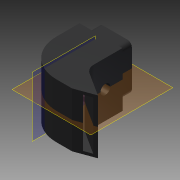
# Autodesk Inventor part: Tobera_05
Saved by Autodesk Inventor 2015 (Build 190159000, 159)
## iProperties
Created: 2013-03-26
Part Number: Tobera_05
Document SubType Name: Modeling
Designer: Lukas
Density: 1 g/cm^3
Mass: 3.92133 g
Surface Area: 46.33 cm^2
Volume: 3.92133 cm^3
Material: Generic
Appearance: Rubber - Black - Version 1.1
Author: Lukas
Autodesk Inventor part; units mm, degrees
ref_plane "YZ Plane" through (0, 0, 0) normal (1, 0, 0) x (0, 1, 0)
ref_plane "XZ Plane" through (0, 0, 0) normal (0, 1, 0) x (-1, 0, 0)
sketch "Boceto1" plane through (0, 0, 0) normal (0, 0, 1) x (1, 0, 0)
  line L0 (-15, 0) -> (0, 0)
  line L1 (0, 0) -> (0, -10)
  arc A0 (0, -10) -> (1.8389, -13.3659) centre (4, -10) ccw
  line L2 (3.4222, -21) -> (-2, -21)
  arc A1 (-15, -8) -> (-2, -21) centre (-2, -8) ccw
  line L3 (-15, -8) -> (-15, 0)
  line L4 (1.8389, -13.3659) -> (10, -18.6059)
  line L5 (10, -18.6059) -> (3.4222, -21)
  dimension "d0" = 15
  dimension "d1" = 10
  dimension "d2" = 21
  dimension "d9" = 13
  dimension "d106" = 10
  dimension "d107" = 4
  dimension "d108" = 7
  dimension "d109" = 20
  constraints: 12 end point, 4 point on circle, 4 tangent, 2 centre point, 2 perpendicular, 1 coincident, 1 horizontal, 1 parallel
  measures "d0" distance of L0.start L0.end
  measures "d1" distance of L0.end L1.end
  measures "d2" distance between parallel lines of L2 L0
  measures "d9" radius of A1
  measures "d106" distance from line of L1 L4.end
  measures "d107" radius of A0
  measures "d108" distance of L4.end L2.start
  measures "d109" angle of L2 L5
extrude "Extrusión1" add sketch "Boceto1" along normal mid plane 19
sketch "Boceto2" plane through (-15, -8, 9.5) normal (-1, 0, 0) x (0, 0, 1)
  line L0 (-19, 8) -> (0, 8) projected
  point P0 (-9.5, 2)
  point P1 (-9.5, 8)
  dimension "d10" = 6
  constraints: 1 midpoint, 1 vertical alignment
  measures "d10" distance from line of L0 point (-9.5, 2)
hole "Agujero1" at (-15, -6, 0) direction (1, 0, 0) diameter 3.4 end through all counterbore diameter 6.5 counterbore depth 3.4 clearance for "Tornillo de cabeza hueca DIN EN ISO 4762" size "M3" standard "DIN"
shell "Vaciado1" thickness 1 removed faces 2 at (-10, 0, 3.1667) at (7.8074, -19.4039, -3.1667)
ref_plane "Plano de trabajo2" through (-7.5, -8, 9.5) normal (-1, 0, 0) x (0, 0, 1)
sketch "Boceto9" plane through (-2, -20, -8.5) normal (0, 0, 1) x (1, 0, 0)
  line L0 (-12, 20) -> (1, 20) projected
  line L1 (2, 20) -> (-13, 20) projected
  line L2 (-10, 20) -> (-10, 13.1048)
  line L3 (-1, 20) -> (-1, 13.6609)
  line L4 (2, 10) -> (2, 20) projected
  line L5 (-10, 20) -> (-12, 20)
  line L6 (-1, 20) -> (1, 20)
  line L7 (-13, 20) -> (-13, 12) projected
  arc A0 (-13, 12) -> (0, -1) centre (0, 12) ccw projected
  arc A1 (2, 10) -> (3.8389, 6.6341) centre (6, 10) ccw projected
  line L8 (10.8187, 0.9642) -> (3.2986, 5.7926) projected
  arc A2 (-1, 13.6609) -> (3.2986, 5.7926) centre (8.3505, 13.6609) ccw
  arc A3 (-10, 13.1048) -> (-3.0408, 3.5783) centre (0, 13.1048) ccw
  line L9 (-3.0408, 3.5783) -> (8.1696, 0)
  line L10 (-12, 20) -> (-12, 12) projected
  arc A4 (-12, 12) -> (0, 0) centre (0, 12) ccw projected
  line L11 (-12, 20) -> (-12, 12)
  arc A5 (-12, 12) -> (0, 0) centre (0, 12) ccw
  line L12 (0, 0) -> (8.1696, 0)
  line L13 (3.2986, 5.7926) -> (3.8389, 6.6341)
  line L14 (1, 20) -> (2, 20)
  line L15 (2, 20) -> (2, 10)
  arc A6 (2, 10) -> (3.8389, 6.6341) centre (6, 10) ccw
  dimension "d68" = 3
  dimension "d69" = 3
  dimension "d110" = 10
  dimension "d111" = 15
  constraints: 20 end point, 8 point on circle, 8 tangent, 4 centre point, 4 collinear, 4 perpendicular, 2 concentric, 2 point on line, 1 parallel
  measures "d68" distance from line of L1.end L2
  measures "d69" distance between parallel lines of L4 L3
  measures "d110" radius of A3
  measures "d111" angle of L8 L9
extrude "Extrusión17" add sketch "Boceto9" along normal up to surface (17 mm away)
hole "Agujero4" at (-15, -6, 0) direction (1, 0, 0) diameter 3.4 end through all counterbore diameter 6.5 counterbore depth 3.4 clearance for "Tornillo de cabeza hueca DIN EN ISO 4762" size "M3" standard "DIN"
sketch "Boceto20" plane through (-10.6, -6, 0) normal (1, 0, 0) x (0, 0, -1)
  circle A0 centre (0, 0) radius 4.25 projected
  circle A1 centre (0, 0) radius 2.7 projected
extrude "Extrusión18" [suppressed]
sketch "Boceto21" plane through (-15, 0, -9.5) normal (0, 1, 0) x (1, 0, 0)
  line L0 (15, 0) -> (0, 0) projected
  line L1 (0, -19) -> (15, -19) projected
  line L2 (12, -18) -> (3, -18) projected
  line L3 (3, -1) -> (3, -18) projected
  line L4 (3, -1) -> (12, -1) projected
  line L5 (12, -1) -> (12, -18) projected
  line L6 (3, -2.5) -> (12, -2.5)
  line L7 (3, -16.5) -> (12, -16.5)
  dimension "d125" = 2.5
  dimension "d126" = 2.5
  constraints: 4 end point, 4 point on line, 2 perpendicular
  measures "d125" distance between parallel lines of L0 L6
  measures "d126" distance between parallel lines of L1 L7
extrude "Extrusión19" add sketch "Boceto21" against normal blind 5 contours L2 L3 L7 L5 | L6 L3 L4 L5
sketch "Boceto22" plane through (-15, 0, -9.5) normal (0, 1, 0) x (1, 0, 0)
  line L0 (3, -2.5) -> (3, -16.5) projected
  line L1 (3, -2.5) -> (12, -2.5) projected
  line L2 (12, -2.5) -> (12, -16.5) projected
  line L3 (12, -16.5) -> (3, -16.5) projected
  line L4 (1.75, -1.6) -> (13.25, -1.6)
  line L5 (13.25, -1.6) -> (13.25, -17.4)
  line L6 (13.25, -17.4) -> (1.75, -17.4)
  line L7 (1.75, -17.4) -> (1.75, -1.6)
  dimension "d129" = 0.9
  dimension "d130" = 1.25
  dimension "d131" = 1.25
  dimension "d132" = 0.9
  constraints: 8 end point, 2 parallel, 1 horizontal, 1 perpendicular
  measures "d129" distance between parallel lines of L1 L4
  measures "d130" distance between parallel lines of L7 L0
  measures "d131" distance between parallel lines of L5 L2
  measures "d132" distance between parallel lines of L6 L3
extrude "Extrusión20" add sketch "Boceto22" along normal blind 5
sketch "Boceto23" plane through (-13.25, 0, -7.9) normal (-1, 0, 0) x (0, 0, 1)
  line L0 (0, 0) -> (0, 5) projected
  line L1 (15.8, 0) -> (15.8, 5) projected
  line L2 (-1.6, 5) -> (-1.6, 2)
  line L3 (-1.6, 2) -> (-0.1, 3.5)
  line L4 (-0.1, 3.5) -> (-1.6, 5)
  line L5 (-1.6, 0) -> (-1.6, -8) projected
  dimension "d135" = 0.1
  dimension "d136" = 3
  constraints: 6 end point, 1 horizontal alignment, 1 parallel, 1 perpendicular, 1 vertical alignment
  measures "d135" distance from line of L0 L3.end
  measures "d136" distance of L2.start L2.end
extrude "Extrusión21" [suppressed]
fillet "Empalme8" radius 1.5 4 edges at (-13.25, 2.5, 7.9) (-1.75, 2.5, 7.9) (-1.75, 2.5, -7.9) (-13.25, 2.5, -7.9)
move faces "Desplazar cara4" translate (1, 0, 0) faces at (-10.6, -5.661, 3.6922)
sketch "Boceto24" plane through (-7.5, -8, 9.5) normal (-1, 0, 0) x (0, 0, 1)
  line L0 (-17.4, 13) -> (-17.4, 8) projected
  line L1 (-19, 8) -> (0, 8) projected
  line L2 (-19, 11) -> (-19, 13)
  line L3 (-19, 13) -> (-17.4, 13)
  line L4 (-17.4, 13) -> (-17.4, 12.6)
  line L5 (-17.4, 12.6) -> (-19, 11)
  dimension "d143" = 2
  dimension "d146" = 0.4
  constraints: 8 end point, 2 perpendicular, 1 point on line, 1 vertical alignment
  measures "d143" distance of L2.start L2.end
  measures "d146" distance of L0.start L4.end
equation "\"d126\" = d125"
equation "\"d131\" = d130"
equation "\"d132\" = d129"
body "Solid1"
